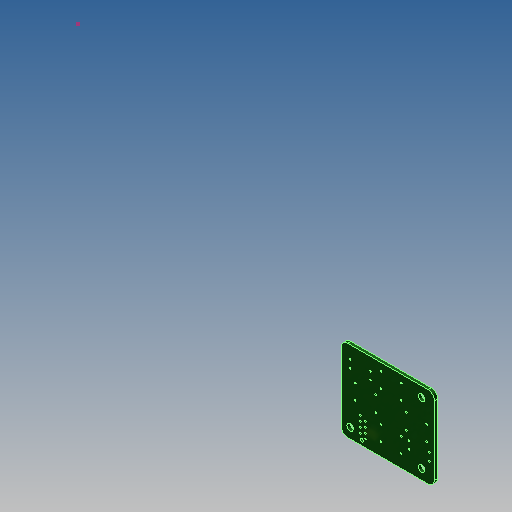
# Autodesk Inventor part: manette_2019_boutons.kicad_pcb_Contour
Saved by Autodesk Inventor 2019 (Build 230136000, 136)
## iProperties
Created: 2019-05-20
Part Number: manette_2019_boutons.kicad_pcb_Contour
Project: Nom Projet
Material: .
Description: Nom pièce
Document SubType Name: Modeling
Designer: Adel.KAHRIMANOVIC
Authority: brut Ø
Density: 0.001 g/cm^3
Appearance: Contour du circuit imprimé
Author: Adel.KAHRIMANOVIC
Material number: ---
Autodesk Inventor part; units mm, degrees
ref_plane "Plan YZ" through (0, 0, 0) normal (1, 0, 0) x (0, 1, 0)
ref_plane "Plan XZ" through (0, 0, 0) normal (0, 1, 0) x (-1, 0, 0)
ref_plane "Plan XY" through (0, 0, 0) normal (0, 0, 1) x (1, 0, 0)
sketch "Esquisse1" plane through (0, 0, 0) normal (0, 0, 1) x (1, 0, 0)
  point P0 (0, 0)
sketch "Esquisse6" plane through (0, 0, 0) normal (0, 0, 1) x (1, 0, 0)
  arc A0 (135.89, -68.58) -> (132.715, -71.755) centre (135.89, -71.755) ccw
  line L0 (132.715, -71.755) -> (132.715, -106.045)
  arc A1 (132.715, -106.045) -> (135.89, -109.22) centre (135.89, -106.045) ccw
  line L1 (135.89, -109.22) -> (175.895, -109.22)
  arc A2 (175.895, -109.22) -> (179.07, -106.045) centre (175.895, -106.045) ccw
  line L2 (179.07, -106.045) -> (179.07, -71.755)
  arc A3 (179.07, -71.755) -> (175.895, -68.58) centre (175.895, -71.755) ccw
  line L3 (175.895, -68.58) -> (135.89, -68.58)
  circle A4 centre (142.24, -96.52) radius 0.4
  circle A5 centre (144.78, -97.79) radius 0.4
  circle A6 centre (142.24, -99.06) radius 0.4
  circle A7 centre (144.78, -100.33) radius 0.4
  circle A8 centre (142.24, -101.6) radius 0.4
  circle A9 centre (144.78, -102.87) radius 0.4
  circle A10 centre (142.24, -104.14) radius 0.4
  circle A11 centre (144.78, -105.41) radius 0.4
  circle A12 centre (137.16, -78.74) radius 0.4
  circle A13 centre (147.32, -78.74) radius 0.4
  circle A14 centre (166.37, -99.06) radius 0.4
  circle A15 centre (176.53, -99.06) radius 0.4
  circle A16 centre (176.53, -95.25) radius 0.4
  circle A17 centre (166.37, -95.25) radius 0.4
  circle A18 centre (147.32, -74.93) radius 0.4
  circle A19 centre (137.16, -74.93) radius 0.4
  circle A20 centre (149.86, -83.82) radius 0.4
  circle A21 centre (139.7, -83.82) radius 0.4
  circle A22 centre (149.86, -91.44) radius 0.4
  circle A23 centre (139.7, -91.44) radius 0.4
  circle A24 centre (162.56, -95.25) radius 0.4
  circle A25 centre (152.4, -95.25) radius 0.4
  circle A26 centre (162.56, -102.87) radius 0.4
  circle A27 centre (152.4, -102.87) radius 0.4
  circle A28 centre (175.26, -83.82) radius 0.4
  circle A29 centre (165.1, -83.82) radius 0.4
  circle A30 centre (175.26, -91.44) radius 0.4
  circle A31 centre (165.1, -91.44) radius 0.4
  circle A32 centre (162.56, -72.39) radius 0.4
  circle A33 centre (152.4, -72.39) radius 0.4
  circle A34 centre (162.56, -80.01) radius 0.4
  circle A35 centre (152.4, -80.01) radius 0.4
  circle A36 centre (142.98, -106.81) radius 0.75
  circle A37 centre (137.16, -104.14) radius 1.6
  circle A38 centre (172.72, -104.14) radius 1.6
  circle A39 centre (172.72, -73.66) radius 1.6
  constraints: 40 centre point, 8 end point, 8 point on circle
extrude "manette_2019_boutons.kicad_pcb_Contour" add sketch "Esquisse6" along normal blind 1.6
